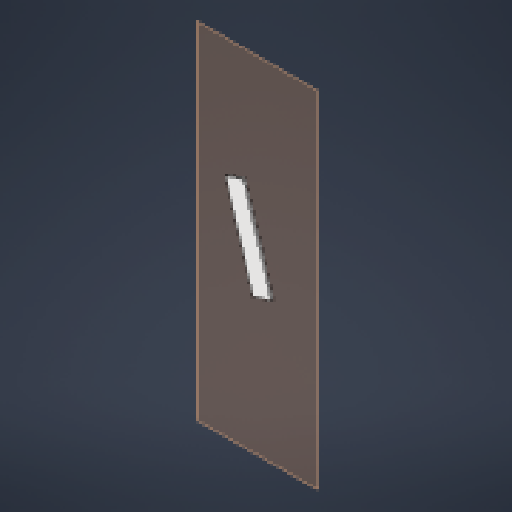
# Autodesk Inventor part: GearBracket
Saved by Autodesk Inventor 2024.3 (Build 283343000, 343)
## iProperties
Created: 2025-03-10
Part Number: GearBracket
Material: Generic
Document SubType Name: Sheet Metal
Designer: jings
Density: 1 g/cm^3
Sheet Metal Rule: Default
Appearance: Default
Author: jings
Autodesk Inventor part; units mm, degrees
ref_plane "YZ Plane" through (0, 0, 0) normal (1, 0, 0) x (0, 1, 0)
ref_plane "XZ Plane" through (0, 0, 0) normal (0, 1, 0) x (-1, 0, 0)
ref_plane "XY Plane" through (0, 0, 0) normal (0, 0, 1) x (1, 0, 0)
ref_plane "Work Plane1" through (231.2168, -695.9876, -158.75) normal (0, 0, 1) x (-0.9997801, -0.0209692, 0)
sketch "Sketch1" plane through (231.2168, -695.9876, -158.75) normal (0, 0, 1) x (-0.9997801, -0.0209692, 0)
  line L0 (191.5805, -690.6559) -> (218.9069, -682.3014)
  line L1 (218.9069, -682.3014) -> (241.1856, -755.1718)
  line L2 (241.1856, -755.1718) -> (213.8592, -763.5264)
  line L3 (213.8592, -763.5264) -> (191.5805, -690.6559)
  arc A0 (211.507, -928.635) -> (222.8439, -923.2276) centre (216.7713, -925.0841) ccw
  line L4 (203.7328, -860.718) -> (222.8439, -923.2276)
  arc A1 (207.9488, -852.7889) -> (203.7328, -860.718) centre (209.8053, -858.8615) ccw
  line L5 (232.2389, -845.3627) -> (207.9488, -852.7889)
  arc A2 (240.168, -849.5787) -> (232.2389, -845.3627) centre (234.0955, -851.4352) ccw
  line L6 (288.8094, -1008.6774) -> (240.168, -849.5787)
  arc A3 (288.8094, -1008.6774) -> (289.6175, -1010.3717) centre (294.8819, -1006.8208) ccw
  line L7 (308.7826, -1038.7851) -> (289.6175, -1010.3717)
  arc A4 (308.7826, -1038.7851) -> (317.5979, -1040.4986) centre (314.047, -1035.2342) ccw
  line L8 (596.6104, -852.3023) -> (317.5979, -1040.4986)
  line L9 (312.5405, -431.1512) -> (596.6104, -852.3023)
  line L10 (95.3316, -577.6604) -> (312.5405, -431.1512)
  arc A5 (95.3316, -577.6604) -> (92.8099, -584.7814) centre (98.8825, -582.9248) ccw
  line L11 (186.4087, -890.9291) -> (92.8099, -584.7814)
  arc A6 (186.4087, -890.9291) -> (187.2168, -892.6234) centre (192.4812, -889.0725) ccw
  line L12 (211.507, -928.635) -> (187.2168, -892.6234)
  line L13 (151.3976, -689.5372) -> (192.5934, -824.2828)
  arc A7 (155.6135, -681.6081) -> (151.3976, -689.5372) centre (157.4701, -687.6806) ccw
  line L14 (179.9037, -674.1818) -> (155.6135, -681.6081)
  arc A8 (187.8328, -678.3978) -> (179.9037, -674.1818) centre (181.7602, -680.2544) ccw
  line L15 (229.0286, -813.1435) -> (187.8328, -678.3978)
  arc A9 (224.8127, -821.0726) -> (229.0286, -813.1435) centre (222.9561, -815) ccw
  line L16 (200.5225, -828.4988) -> (224.8127, -821.0726)
  arc A10 (192.5934, -824.2828) -> (200.5225, -828.4988) centre (198.666, -822.4263) ccw
  arc A11 (140.2582, -653.102) -> (148.1873, -657.3179) centre (146.3307, -651.2454) ccw
  line L17 (122.5952, -595.3289) -> (140.2582, -653.102)
  arc A12 (125.1168, -588.2079) -> (122.5952, -595.3289) centre (128.6677, -593.4723) ccw
  line L18 (147.1366, -573.3554) -> (125.1168, -588.2079)
  arc A13 (156.76, -576.7633) -> (147.1366, -573.3554) centre (150.6874, -578.6198) ccw
  line L19 (176.6934, -641.9626) -> (156.76, -576.7633)
  arc A14 (172.4774, -649.8917) -> (176.6934, -641.9626) centre (170.6209, -643.8192) ccw
  line L20 (148.1873, -657.3179) -> (172.4774, -649.8917)
  line L21 (440.6793, -731.4527) -> (242.0503, -738.1789)
  arc A15 (235.844, -729.7287) -> (242.0503, -738.1789) centre (241.8354, -731.8326) ccw
  line L22 (235.844, -729.7287) -> (312.2467, -512.1467)
  arc A16 (323.7318, -511.066) -> (312.2467, -512.1467) centre (318.238, -514.2505) ccw
  line L23 (323.7318, -511.066) -> (445.9582, -721.9218)
  arc A17 (440.6793, -731.4527) -> (445.9582, -721.9218) centre (440.4644, -725.1063) ccw
  line L24 (293.699, -488.3023) -> (226.6453, -679.2602)
  arc A18 (214.5814, -679.0129) -> (226.6453, -679.2602) centre (220.6539, -677.1564) ccw
  line L25 (214.5814, -679.0129) -> (177.6445, -558.1977)
  arc A19 (180.1661, -551.0767) -> (177.6445, -558.1977) centre (183.717, -556.3411) ccw
  line L26 (180.1661, -551.0767) -> (284.1568, -480.9341)
  arc A20 (293.699, -488.3023) -> (284.1568, -480.9341) centre (287.7077, -486.1985) ccw
  line L27 (338.9686, -980.6315) -> (474.0479, -788.3553)
  arc A21 (484.7375, -788.821) -> (474.0479, -788.3553) centre (479.2438, -792.0056) ccw
  line L28 (484.7375, -788.821) -> (526.8957, -861.5491)
  arc A22 (524.9528, -869.998) -> (526.8957, -861.5491) centre (521.4019, -864.7336) ccw
  line L29 (524.9528, -869.998) -> (347.7154, -989.5462)
  arc A23 (338.9686, -980.6315) -> (347.7154, -989.5462) centre (344.1645, -984.2818) ccw
  line L30 (303.3396, -969.3278) -> (242.8789, -771.57)
  arc A24 (248.7366, -763.3671) -> (242.8789, -771.57) centre (248.9515, -769.7134) ccw
  line L31 (248.7366, -763.3671) -> (452.9866, -756.4505)
  arc A25 (458.3974, -766.4471) -> (452.9866, -756.4505) centre (453.2015, -762.7968) ccw
  line L32 (458.3974, -766.4471) -> (314.608, -971.1215)
  arc A26 (303.3396, -969.3278) -> (314.608, -971.1215) centre (309.4121, -967.4712) ccw
  line L33 (215.2197, -740.1923) -> (205.7566, -709.24)
  line L34 (210.4881, -724.7162) -> (230.0462, -718.7366) construction
  point P0 (216.5716, -700.683)
  dimension "d0" = 76.2
  dimension "d27" = 28.575
  measures "d0" distance of L2.end L0.start
  measures "d27" distance of L0.start L0.end
extrude "Plate1" add sketch "Sketch1" along normal blind 3.048 contours L0 A18 L1 L2 L3 | L0 L1 A18
sketch "Sketch2" plane through (-4.8448, -19.3786, -152.654) normal (-0.9499637, -0.3123604, 0) x (0.3123604, -0.9499637, 0)
  line L0 (-76.2, 0) -> (0, 0)
  line L1 (0, 0) -> (0, 311.404)
  line L2 (0, 311.404) -> (-76.2, 311.404)
  line L3 (-76.2, 311.404) -> (-76.2, 0)
  constraints: 6 end point, 1 horizontal, 1 perpendicular, 1 vertical
edge flange "Flange1" height 317.5 angle 90 thickness 3.048 bend radius 3.048 thickness toward (-0.9499637, -0.3123604, 0) relief tear relief width 3.048 relief depth 1.524 edges at (-13.8502, 17.7671, -155.702) wall of the first edge with corners at (-28.6466, 53.0087, -152.654) (-4.8448, -19.3786, -152.654) (-4.8448, -19.3786, 158.75) (-28.6466, 53.0087, 158.75)
bend "Bend1"
corner "Corner1"
sketch "Sketch3" plane through (-7.7403, -20.3306, 155.702) normal (0, 0, 1) x (1, 0, 0)
  line L0 (-23.8019, 72.3872) -> (0, 0)
  line L1 (0, 0) -> (27.1452, 8.9257)
  line L2 (27.1452, 8.9257) -> (3.3434, 81.3129)
  line L3 (3.3434, 81.3129) -> (-23.8019, 72.3872)
  constraints: 6 end point, 1 perpendicular, 2 other
edge flange "Flange2" height 28.575 angle 90 thickness 3.048 bend radius 3.048 thickness toward (0, 0, 1) relief tear relief width 3.048 relief depth 1.524 edges at (-16.7457, 16.815, 158.75) wall of the first edge with corners at (-31.5421, 52.0566, 155.702) (-7.7403, -20.3306, 155.702) (19.4049, -11.4049, 155.702) (-4.3969, 60.9823, 155.702)
bend "Bend2"
corner "Corner2"
sketch "Sketch4" plane through (-31.5421, 52.0566, 152.654) normal (-0.9499637, -0.3123604, 0) x (0, 0, -1)
  line L0 (-6.096, 80.617) -> (-6.096, -4.417)
  line L1 (-6.096, 38.1) -> (311.404, 38.1) construction
  line L2 (311.404, 74.4136) -> (311.404, 1.7864)
  circle A0 centre (44.704, 38.1) radius 31.75
  circle A1 centre (114.554, 38.1) radius 38.1
  circle A2 centre (190.754, 38.1) radius 38.1
  circle A3 centre (260.604, 38.1) radius 31.75
  circle A4 centre (44.704, 38.1) radius 16.2087 construction
  circle A5 centre (260.604, 38.1) radius 16.2087 construction
  circle A6 centre (44.704, 38.1) radius 14.2875
  circle A7 centre (114.554, 38.1) radius 14.2875
  circle A8 centre (190.754, 38.1) radius 14.2875
  circle A9 centre (260.604, 38.1) radius 14.2875
  line L3 (-6.096, 0) -> (-6.096, 76.2) projected
  line L4 (311.404, 0) -> (311.404, 76.2) projected
  line L5 (44.704, 38.1) -> (-6.096, 38.1) construction
  line L6 (260.604, 38.1) -> (311.404, 38.1) construction
  dimension "d22" = 28.575
  dimension "d23" = 63.5
  dimension "d28" = 76.2
  constraints: 10 centre point, 10 end point, 5 equal radius, 4 coincident, 4 collinear, 4 point on line, 3 midpoint, 3 tangent, 2 concentric, 1 horizontal, 1 perpendicular
  measures "d22" diameter of A7
  measures "d23" diameter of A0
  measures "d28" diameter of A1
extrude "Cut1" cut sketch "Sketch4" against normal blind 3.048 contours A6 | A7 | A8 | A9
equation "\"d25\" = Thickness"
equation "\"d1\" = Thickness"
equation "\"d2\" = BendReliefWidth"
equation "\"d3\" = BendReliefDepth"
equation "\"d4\" = MinimumRemnant"
equation "\"d5\" = TransitionRadius"
equation "\"d8\" = BendRadius"
equation "\"d9\" = CornerReliefSize"
equation "\"d10\" = GapSize"
equation "\"d11\" = JacobiRadiusSize"
equation "\"d12\" = BendReliefWidth"
equation "\"d13\" = BendReliefDepth"
equation "\"d14\" = MinimumRemnant"
equation "\"d15\" = TransitionRadius"
equation "\"d18\" = BendRadius"
equation "\"d19\" = CornerReliefSize"
equation "\"d20\" = GapSize"
equation "\"d21\" = JacobiRadiusSize"
equation "\"BendRadius\" = Thickness"
equation "\"BendReliefWidth\" = Thickness"
equation "\"BendReliefDepth\" = 0.5 * Thickness"
equation "\"CornerReliefSize\" = 4 * Thickness"
equation "\"MinimumRemnant\" = 2 * Thickness"
equation "\"TransitionRadius\" = BendRadius"
equation "\"JacobiRadiusSize\" = BendRadius"
equation "\"GapSize\" = Thickness"
equation "\"Thickness\" = 3.048"
body "Solid1"
